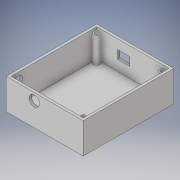
# Autodesk Inventor part: bottom
Saved by Autodesk Inventor 2018.1 (Build 221171000, 171)
## iProperties
Created: 2022-03-02
Part Number: bottom
Material: Generic
Document SubType Name: Modeling
Designer: micha
Density: 1 g/cm^3
Appearance: Default
Author: micha
Autodesk Inventor part; units mm, degrees
ref_plane "YZ Plane" through (0, 0, 0) normal (1, 0, 0) x (0, 1, 0)
ref_plane "XZ Plane" through (0, 0, 0) normal (0, 1, 0) x (-1, 0, 0)
ref_plane "XY Plane" through (0, 0, 0) normal (0, 0, 1) x (1, 0, 0)
sketch "Sketch1" plane through (0, 0, 0) normal (0, 1, 0) x (-1, 0, 0)
  line L0 (0, 0) -> (63, 0)
  line L1 (63, 0) -> (63, -74)
  line L2 (63, -74) -> (0, -74)
  line L3 (0, -74) -> (0, 0)
  dimension "d0" = 63
  dimension "d1" = 74
  constraints: 8 end point, 2 parallel, 1 horizontal, 1 perpendicular
  measures "d0" distance of L1.end L2.end
  measures "d1" distance of L0.end L1.end
extrude "Extrusion1" add sketch "Sketch1" along normal blind 25
sketch "Sketch2" plane through (0, 25, 0) normal (0, 1, 0) x (1, 0, 0)
  line L0 (-2, 2) -> (-61, 2)
  line L1 (-61, 2) -> (-61, 72)
  line L2 (-61, 72) -> (-2, 72)
  line L3 (-2, 72) -> (-2, 2)
  line L4 (-63, 74) -> (-63, 0) projected
  line L5 (-63, 0) -> (0, 0) projected
  line L6 (0, 0) -> (0, 74) projected
  dimension "d5" = 70
  dimension "d6" = 2
  dimension "d7" = 59
  dimension "d8" = 2
  constraints: 8 end point, 2 parallel, 1 horizontal, 1 perpendicular
  measures "d5" distance of L0.end L1.end
  measures "d6" distance between parallel lines of L5 L0
  measures "d7" distance of L1.end L2.end
  measures "d8" distance between parallel lines of L3 L6
extrude "Extrusion2" cut sketch "Sketch2" against normal blind 23
sketch "Sketch3" plane through (0, 0, -74) normal (0, 0, -1) x (-1, 0, 0)
  line L0 (44, 17.5) -> (34, 17.5)
  line L1 (34, 17.5) -> (34, 10.5)
  line L2 (34, 10.5) -> (44, 10.5)
  line L3 (44, 10.5) -> (44, 17.5)
  line L4 (63, 0) -> (63, 25) projected
  line L5 (0, 25) -> (63, 25) projected
  point P0 (0, 0)
  dimension "d11" = 10
  dimension "d12" = 7
  dimension "d13" = 19
  dimension "d21" = 7.5
  constraints: 8 end point, 2 parallel, 1 horizontal, 1 perpendicular
  measures "d11" distance of L2.end L1.end
  measures "d12" distance of L1.end L0.end
  measures "d13" distance between parallel lines of L4 L3
  measures "d21" distance between parallel lines of L5 L0
extrude "Extrusion3" cut sketch "Sketch3" against normal up to next
sketch "Sketch4" plane through (-63, 0, -74) normal (-1, 0, 0) x (0, 0, 1)
  circle A0 centre (66, 19) radius 3.25
  line L0 (74, 0) -> (74, 25) projected
  line L1 (0, 25) -> (74, 25) projected
  dimension "d16" = 6.5
  dimension "d17" = 8
  dimension "d18" = 6
  constraints: 1 centre point
  measures "d16" diameter of A0
  measures "d17" distance from line of L0 A0.centre
  measures "d18" distance from line of A0.centre L1
extrude "Extrusion4" cut sketch "Sketch4" against normal up to next
sketch "Sketch5" plane through (-63, 0, 0) normal (0, 0, 1) x (1, 0, 0)
  circle A0 centre (23, 19) radius 4.25
  line L0 (29, 17.5) -> (29, 10.5) projected
  line L1 (0, 25) -> (63, 25) projected
  point P0 (63, 0)
  dimension "d22" = 8.5
  dimension "d23" = 6
  dimension "d24" = 6
  constraints: 1 centre point
  measures "d22" diameter of A0
  measures "d23" distance from line of A0.centre L0
  measures "d24" distance from line of L1 A0.centre
extrude "Extrusion5" cut sketch "Sketch5" against normal up to next
sketch "Sketch6" plane through (0, 2, 0) normal (0, 1, 0) x (1, 0, 0)
  circle A0 centre (-4.5, 4.5) radius 2.5
  line L0 (0, 0) -> (0, 74) projected
  line L1 (-63, 0) -> (0, 0) projected
  circle A1 centre (-4.5, 69.5) radius 2.5
  line L2 (0, 74) -> (-63, 74) projected
  circle A2 centre (-58.5, 69.5) radius 2.5
  line L3 (-63, 74) -> (-63, 0) projected
  dimension "d27" = 5
  dimension "d28" = 4.5
  dimension "d29" = 4.5
  dimension "d30" = 5
  dimension "d31" = 4.5
  dimension "d32" = 5
  dimension "d33" = 4.5
  constraints: 3 centre point
  measures "d27" diameter of A0
  measures "d28" distance from line of L0 A0.centre
  measures "d29" distance from line of L1 A0.centre
  measures "d30" diameter of A1
  measures "d31" distance from line of L2 A1.centre
  measures "d32" diameter of A2
  measures "d33" distance from line of A2.centre L3
extrude "Extrusion6" add sketch "Sketch6" along normal blind 21 contours A0 | A1 | A2
sketch "Sketch7" plane through (0, 23, 0) normal (0, 1, 0) x (1, 0, 0)
  arc A0 (-61, 69.5) -> (-58.5, 72) centre (-58.5, 69.5) ccw projected
  arc A1 (-4.5, 72) -> (-2, 69.5) centre (-4.5, 69.5) ccw projected
  arc A2 (-4.5, 72) -> (-2, 69.5) centre (-4.5, 69.5) ccw projected
  line L0 (-58.5, 72) -> (-4.5, 72) projected
  arc A3 (-61, 69.5) -> (-58.5, 72) centre (-58.5, 69.5) ccw projected
  line L1 (-61, 2) -> (-61, 69.5) projected
  line L2 (-4.5, 2) -> (-61, 2) projected
  arc A4 (-2, 4.5) -> (-4.5, 2) centre (-4.5, 4.5) ccw projected
  line L3 (-2, 69.5) -> (-2, 4.5) projected
  circle A5 centre (-4.5, 69.5) radius 1.5
  circle A6 centre (-58.5, 69.5) radius 1.5
  circle A7 centre (-4.5, 4.5) radius 1.5
  point P0 (0, 0)
  dimension "d36" = 3
  dimension "d37" = 3
  dimension "d38" = 3
  constraints: 3 centre point, 3 coincident
  measures "d36" diameter of A5
  measures "d37" diameter of A6
  measures "d38" diameter of A7
extrude "Extrusion7" cut sketch "Sketch7" against normal blind 19 contours A5 | A6 | A7
sketch "Sketch8" plane through (0, 2, 0) normal (0, 1, 0) x (1, 0, 0)
  arc A0 (-4.5, 2) -> (-2, 4.5) centre (-4.5, 4.5) ccw projected
  line L0 (-4.5, 2) -> (-2, 2)
  line L1 (-2, 2) -> (-2, 4.5)
  line L2 (-2, 4.5) -> (-2, 4.1991)
  arc A1 (-4.5, 2) -> (-2, 4.5) centre (-4.5, 4.5) ccw
  arc A2 (-4.5, 72) -> (-2, 69.5) centre (-4.5, 69.5) ccw projected
  line L3 (-4.5, 72) -> (-2, 72)
  arc A3 (-2, 69.5) -> (-4.5, 72) centre (-4.5, 69.5) ccw projected
  line L4 (-2, 72) -> (-2, 69.5)
  arc A4 (-2, 69.5) -> (-4.5, 72) centre (-4.5, 69.5) ccw
  arc A5 (-58.5, 72) -> (-61, 69.5) centre (-58.5, 69.5) ccw projected
  arc A6 (-58.5, 72) -> (-61, 69.5) centre (-58.5, 69.5) ccw
  line L5 (-61, 69.5) -> (-61, 72)
  line L6 (-61, 72) -> (-58.5, 72)
  point P0 (0, 0)
  constraints: 14 end point, 6 point on circle, 6 tangent, 3 centre point, 3 perpendicular, 2 horizontal, 1 concentric, 1 point on line, 1 vertical
extrude "Extrusion8" add sketch "Sketch8" along normal blind 21 contours A0 L1 L0 | L3 L4 A3 | A5 L5 L6
body "Solid1"
